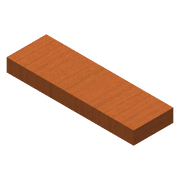
# Autodesk Inventor part: 2p3ph
Saved by Autodesk Inventor 2016 SP2 (Build 200236200, 236)
## iProperties
Company: HERA Project
Created: 2013-09-06
Part Number: 2p3ph
Material: Wood (Cherry)
Document SubType Name: Modeling
Designer: David DeBoer
Density: 0.5 g/cm^3
Mass: 635.373 g
Surface Area: 1042.45 cm^2
Volume: 1270.75 cm^3
Description: post horizontal holder
Appearance: Cherry - Natural Low Gloss
Author: David DeBoer
Autodesk Inventor part; units mm, degrees
ref_plane "YZ Plane" through (0, 0, 0) normal (1, 0, 0) x (0, 1, 0)
ref_plane "XZ Plane" through (0, 0, 0) normal (0, 1, 0) x (-1, 0, 0)
ref_plane "XY Plane" through (0, 0, 0) normal (0, 0, 1) x (1, 0, 0)
sketch "Sketch1" plane through (0, 0, 0) normal (0, 0, 1) x (1, 0, 0)
  line L0 (0, 0) -> (365, 0)
  line L1 (0, 0) -> (0, 38)
  line L2 (0, 38) -> (365, 38)
  line L3 (365, 0) -> (365, 38)
  dimension "d0" = 365
  dimension "d1" = 38
  dimension "d2" = 90
  constraints: 8 end point, 2 perpendicular
  measures "d0" distance of L0.start L0.end
  measures "d1" distance of L0.start L1.end
  measures "d2" angle of L3 L0
extrude "Extrusion1" add sketch "Sketch1" along normal blind 114
body "Solid1"
